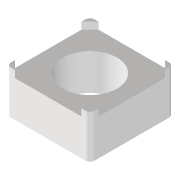
# Autodesk Inventor part: 00_VCM_M12
Saved by Autodesk Inventor 2022 (Build 260153000, 153)
## iProperties
Created: 2023-01-02
Part Number: 00_VCM_M12
Material: Generisch
Document SubType Name: Modeling
Designer: diederichbenedict
Density: 1 g/cm^3
Appearance: Vorgabe
Author: diederichbenedict
Autodesk Inventor part; units mm, degrees
ref_plane "YZ Plane" through (0, 0, 0) normal (1, 0, 0) x (0, 1, 0)
ref_plane "XZ Plane" through (0, 0, 0) normal (0, 1, 0) x (-1, 0, 0)
ref_plane "XY Plane" through (0, 0, 0) normal (0, 0, 1) x (1, 0, 0)
sketch "Skizze1" plane through (0, 0, 0) normal (0, 1, 0) x (-1, 0, 0)
  line L0 (-9, -9) -> (9, -9)
  line L1 (9, -9) -> (9, 9)
  line L2 (9, 9) -> (-9, 9)
  line L3 (-9, 9) -> (-9, -9)
  line L4 (-9, -9) -> (9, 9) construction
  line L5 (9, -9) -> (-9, 9) construction
  circle A0 centre (0, 0) radius 5.8
  dimension "d0" = 18
  dimension "d1" = 18
  dimension "d2" = 11.6
  constraints: 12 end point, 2 midpoint, 2 parallel, 1 centre point, 1 coincident, 1 horizontal, 1 perpendicular
  measures "d0" distance of L2.end L1.end
  measures "d1" distance of L1.end L0.end
  measures "d2" diameter of A0
extrude "Extrusion1" add sketch "Skizze1" along normal blind 7.8
sketch "Skizze2" plane through (0, 7.8, 0) normal (0, 1, 0) x (1, 0, 0)
  line L0 (-9, 9) -> (-9, -9) projected
  line L1 (-9, -9) -> (9, -9) projected
  line L2 (9, -9) -> (9, 9) projected
  line L3 (9, 9) -> (-9, 9) projected
  circle A0 centre (0, 0) radius 5.8 projected
  line L4 (-9, 9) -> (-9, -9) projected
  line L5 (-9, -7.1615) -> (-7.1615, -9)
  line L6 (-9, -7.1615) -> (-6.4, -7.1615) construction
  dimension "d5" = 45
  dimension "d6" = 1.3
  constraints: 4 end point, 2 point on line, 1 equal length, 1 horizontal
  measures "d5" angle of L5 L6
  measures "d6" distance from line of L5 L0.end
extrude "Extrusion2" add sketch "Skizze2" along normal blind 1.5 contours L5 L1 L0
pattern_circular "Runde Anordnung1" count 4 over 360 about axis through (0, 0, 0) along (0, 1, 0) of "Extrusion2"
fillet "Rundung1" radius 1 4 edges at (-9, 4.65, 9) (9, 4.65, 9) (9, 4.65, -9) (-9, 4.65, -9)
